Autodesk Fusion 360 part; units mm, degrees
(part 2 of 2)
extrude "Extrude34" add 1 faces at (-31.175, -16.675, -1.0583) along direction (-1, 0, 0) blind 3 separate body on bodies 2 makes body 17
combine "Combine12" operation add target body 2 tool bodies 16 17
combine "Combine13" operation cut target body 2 tool bodies 5 8 4 3 keep tools
sketch "cover" plane through (0, 0, 25) normal (0, 0, 1) x (1, 0, 0)
  line L0 (-31.175, 46.825) -> (-31.175, -48.425)
  line L1 (-31.175, -48.425) -> (-28, -48.425)
  line L2 (-28, -48.425) -> (-28, 46.825)
  line L3 (-28, 46.825) -> (-31.175, 46.825)
  line L4 (-28, 46.825) -> (-28, 40.65)
  line L5 (-28, 40.65) -> (-29.5875, 40.65)
  line L6 (-29.5875, 40.65) -> (27.9875, 40.65)
  line L7 (27.9875, 40.65) -> (27.9875, -45.425)
  line L8 (27.9875, -45.425) -> (-29.5875, -45.425)
  line L9 (-29.5875, -45.425) -> (-29.5875, 40.65)
  dimension "d152" = 6.175
  dimension "d153" = 1.5875
  dimension "d154" = 57.575
  dimension "d155" = 86.075
  constraint coincident L2.end L3.start
  constraint perpendicular L3 L4
  constraint perpendicular L0 L5
  constraint horizontal L6
  constraint vertical L7
  constraint horizontal L8
  constraint vertical L9
  measures "d152" distance of L2.end L4.end
  measures "d153" distance of L4.end L5.end
  measures "d154" distance of L5.end L6.end
  measures "d155" distance of L5.end L8.end
extrude "Extrude35" add sketch "cover" against normal blind 3.175 separate body contours L2 L6 L7 L8 makes body 18
extrude "Extrude36" add 1 faces at (-28, -16.7333, 22.8833) along direction (-1, 0, 0) blind 1.588 separate body on bodies 18 makes body 19
combine "Combine14" operation add target body 18 tool bodies 19
move_body "Move7" bodies 18 to x (1, 0, 0) y (0, 1, 0) z (0, 0, 1) at (0, 0, -3)
extrude "Extrude37" cut 1 faces at (-31.175, 42.7667, 20.7667) along direction (1, 0, 0) blind 3.175 on bodies 8 bodies 8
extrude "Extrude38" cut 1 faces at (29.575, 42.7667, 20.7667) along direction (-1, 0, 0) blind 3.175 on bodies 8 bodies 8
extrude "Extrude39" add 1 faces at (-30.1167, 43.825, 19.5333) along direction (0, -1, 0) blind 3.175 separate body on bodies 5 makes body 20
combine "Combine15" operation add target body 20 tool bodies 5
extrude "Extrude40" add 1 faces at (28.5167, 43.825, 19.5333) along direction (0, -1, 0) blind 3.175 separate body on bodies 4 makes body 21
combine "Combine16" operation add target body 21 tool bodies 4
extrude "Extrude41" add 1 faces at (-30.1167, 42.7667, 6.7) along direction (0, 0, 1) blind 7 on bodies 8 bodies 8
extrude "Extrude42" add 1 faces at (28.5167, 41.7083, 6.7) along direction (0, 0, 1) blind 7 separate body on bodies 8 makes body 22
combine "Combine17" operation add target body 22 tool bodies 8
combine "Combine18" operation cut target body 21 tool bodies 22 keep tools
combine "Combine19" operation cut target body 20 tool bodies 22 keep tools
extrude "Extrude43" add 1 faces at (8.7957, -45.425, 19.8833) along direction (0, -1, 0) blind 3 separate body on bodies 18 makes body 23
combine "Combine20" operation add target body 18 tool bodies 23
combine "Combine21" operation cut target body 20 tool bodies 18 keep tools
combine "Combine22" operation cut target body 21 tool bodies 18 keep tools
sketch "Sketch21" plane through (0, 0, 9.7) normal (0, 0, 1) x (1, 0, 0)
  line L0 (-28, -42.25) -> (-28, -45.425)
  line L1 (-28, -45.425) -> (26.4, -45.425)
  line L2 (26.4, -45.425) -> (26.4, -42.25)
  line L3 (26.4, -42.25) -> (-28, -42.25)
  line L4 (26.4, -45.425) -> (10, -45.425)
  line L5 (10, -45.425) -> (10, -42.25)
  line L6 (10, -42.25) -> (26.4, -42.25)
  line L7 (26.4, -42.25) -> (26.4, -45.425)
  line L8 (-28, -45.425) -> (-10, -45.425)
  line L9 (-10, -45.425) -> (-10, -42.25)
  line L10 (-10, -42.25) -> (-28, -42.25)
  line L11 (-28, -42.25) -> (-28, -45.425)
  dimension "d174" = 16.4
  dimension "d175" = 3.175
  dimension "d176" = 18
  dimension "d177" = 3.175
  constraint horizontal L4
  constraint vertical L5
  constraint horizontal L6
  constraint vertical L7
  constraint coincident L1.end L2.start
  constraint horizontal L8
  constraint vertical L9
  constraint horizontal L10
  constraint vertical L11
  constraint coincident L0.end L1.start
  measures "d174" distance of L1.end L4.end
  measures "d175" distance of L1.end L2.end
  measures "d176" distance of L0.end L8.end
  measures "d177" distance of L0.end L0.start
extrude "Extrude44" add sketch "Sketch21" along normal blind 9.125 separate body contours L0 L1 L3 L8 L9 L10 L11 makes body 24
extrude "Extrude45" add sketch "Sketch21" along normal blind 9.125 separate body contours L1 L2 L3 L4 L5 L6 L7 makes body 25
combine "Combine23" operation add target body 24 tool bodies 3 25
extrude "Extrude46" add 1 faces at (-30.1167, -43.3083, 6.7) along direction (0, 0, 1) blind 5 on bodies 24 bodies 24
extrude "Extrude47" add 1 faces at (28.5167, -44.3667, 6.7) along direction (0, 0, 1) blind 5 on bodies 24 bodies 24
combine "Combine24" operation cut target body 20 tool bodies 24 keep tools
combine "Combine25" operation cut target body 21 tool bodies 24 keep tools
extrude "Extrude48" cut 1 faces at (8.7957, -48.425, 19.8833) along direction (0, 1, 0) blind 3 on bodies 18 bodies 18
sketch "Sketch22" plane through (0, -45.425, 0) normal (0, -1, 0) x (1, 0, 0)
  line L0 (27.9875, 22) -> (-29.588, 22)
  line L1 (-29.588, 22) -> (-29.588, 18.825)
  line L2 (-29.588, 18.825) -> (27.9875, 18.825)
  line L3 (27.9875, 18.825) -> (27.9875, 22)
  line L4 (27.9875, 18.825) -> (9.9995, 18.825)
  line L5 (9.9995, 18.825) -> (-10.0005, 18.825)
  line L6 (-10.0005, 18.825) -> (-10.0005, 22)
  line L7 (-10.0005, 22) -> (9.9995, 22)
  line L8 (9.9995, 22) -> (9.9995, 18.825)
  dimension "d188" = 17.988
  dimension "d189" = 20
  dimension "d190" = 3.175
  constraint coincident L2.end L3.start
  constraint perpendicular L3 L4
  constraint horizontal L5
  constraint vertical L6
  constraint horizontal L7
  constraint vertical L8
  measures "d188" distance of L2.end L4.end
  measures "d189" distance of L4.end L5.end
  measures "d190" distance of L4.end L7.end
extrude "Extrude49" cut sketch "Sketch22" against normal blind 21.6 contours L0 L2 L5 L6 L7 L8 bodies 18
extrude "Extrude50" cut 1 faces at (-3.3338, -23.825, 20.9417) along direction (0, 1, 0) blind 3.175 on bodies 18 bodies 18
extrude "Extrude51" cut 1 faces at (27.4583, 15.075, 25) along direction (0, 0, -1) blind 6.175 on bodies 21 bodies 21
extrude "Extrude52" add 1 faces at (28.5167, 15.075, 18.825) along direction (0, 0, 1) blind 6.175 separate body on bodies 21 makes body 26
combine "Combine26" operation add target body 21 tool bodies 26
extrude "Extrude53" cut 1 faces at (-30.1167, 15.075, 25) along direction (0, 0, -1) blind 6.175 on bodies 20 bodies 20
extrude "Extrude54" add 1 faces at (-30.1167, 15.075, 18.825) along direction (0, 0, 1) blind 6.175 separate body on bodies 20 makes body 27
combine "Combine27" operation add target body 27 tool bodies 20
sketch "lockers" plane through (-31.175, 0, 0) normal (-1, 0, 0) x (0, 0, 1)
  line L0 (11.7, -45.425) -> (3, -45.425)
  line L1 (3, -45.425) -> (3, -42.25)
  line L2 (3, -42.25) -> (11.7, -42.25)
  line L3 (11.7, -42.25) -> (11.7, -45.425)
  line L4 (13.7, 40.65) -> (3, 40.65)
  line L5 (3, 40.65) -> (3, 43.825)
  line L6 (3, 43.825) -> (13.7, 43.825)
  line L7 (13.7, 43.825) -> (13.7, 40.65)
  line L8 (0, -48.425) -> (25, -48.425)
  line L9 (25, -48.425) -> (25, 46.825)
  line L10 (25, 46.825) -> (0, 46.825)
  line L11 (0, 46.825) -> (0, 15)
  line L12 (0, 15) -> (-3.175, 15)
  line L13 (-3.175, 15) -> (-3.175, -15)
  line L14 (-3.175, -15) -> (0, -15)
  line L15 (0, -15) -> (0, -48.425)
  line L16 (0, 0) -> (10, 0)
  line L17 (10, 0) -> (13.175, 0)
  line L18 (13.175, 0) -> (13.175, 5)
  line L19 (13.175, 5) -> (10, 5)
  line L20 (10, 5) -> (10, 0)
  dimension "d203" = 10
  dimension "d204" = 3.175
  dimension "d205" = 5
  constraint coincident L16.start origin
  constraint horizontal L16
  constraint horizontal L17
  constraint vertical L18
  constraint horizontal L19
  constraint vertical L20
  measures "d203" distance of L16.start L16.end
  measures "d204" distance of L16.end L17.end
  measures "d205" distance of L16.end L19.end
extrude "Extrude55" add sketch "lockers" against normal blind 8.175 separate body contours L17 L18 L19 L20 makes body 28
extrude "Extrude56" add 1 faces at (-23, 3.3333, 11.0583) along direction (1, 0, 0) blind 1.6 separate body on bodies 28 makes body 29
combine "Combine28" operation add target body 28 tool bodies 29
combine "Combine29" operation cut target body 27 tool bodies 28 keep tools
copy_body "CopyPasteBodies8" bodies 28 makes body 30
move_body "Move9" bodies 30 to x (1, 0, 0) y (0, 1, 0) z (0, 0, 1) at (50.975, 0, 0)
extrude "Extrude57" cut 1 faces at (19.8, 3.3333, 11.0583) along direction (1, 0, 0) blind 1.6 on bodies 30 bodies 30
combine "Combine30" operation cut target body 21 tool bodies 30 keep tools
extrude "Extrude58" cut 1 faces at (-29.588, -16.7333, 20.9417) along direction (1, 0, 0) blind 1.588 on bodies 18 bodies 18
extrude "Extrude59" cut 1 faces at (27.9875, -16.7333, 20.9417) along direction (-1, 0, 0) blind 1.588 on bodies 18 bodies 18
sketch "Sketch28" plane through (0, 40.65, 0) normal (0, 1, 0) x (-1, 0, 0)
  line L0 (-26.3995, 22) -> (-26.3995, 18.825)
  line L1 (-26.3995, 18.825) -> (28, 18.825)
  line L2 (28, 18.825) -> (28, 22)
  line L3 (28, 22) -> (-26.3995, 22)
  line L4 (-26.3995, 18.825) -> (-21.6995, 18.825)
  line L5 (-21.6995, 18.825) -> (-14.6995, 18.825)
  line L6 (-14.6995, 18.825) -> (-14.6995, 22)
  line L7 (-14.6995, 22) -> (-21.6995, 22)
  line L8 (-21.6995, 22) -> (-21.6995, 18.825)
  line L9 (28, 18.825) -> (21.7, 18.825)
  line L10 (21.7, 18.825) -> (14.7, 18.825)
  line L11 (14.7, 18.825) -> (14.7, 22)
  line L12 (14.7, 22) -> (21.7, 22)
  line L13 (21.7, 22) -> (21.7, 18.825)
  dimension "d216" = 4.7
  dimension "d217" = 7
  dimension "d218" = 3.175
  dimension "d219" = 6.3
  dimension "d220" = 7
  dimension "d221" = 3.175
  constraint coincident L0.end L1.start
  constraint perpendicular L0 L4
  constraint horizontal L5
  constraint vertical L6
  constraint horizontal L7
  constraint vertical L8
  constraint coincident L1.end L2.start
  constraint perpendicular L2 L9
  constraint horizontal L10
  constraint vertical L11
  constraint horizontal L12
  constraint vertical L13
  measures "d216" distance of L0.end L4.end
  measures "d217" distance of L4.end L5.end
  measures "d218" distance of L4.end L7.end
  measures "d219" distance of L1.end L9.end
  measures "d220" distance of L9.end L10.end
  measures "d221" distance of L9.end L12.end
extrude "Extrude60" add sketch "Sketch28" along normal blind 3.175 contours L1 L3 L5 L6 L7 L8 bodies 18
extrude "Extrude61" add sketch "Sketch28" along normal blind 3.175 contours L1 L3 L10 L11 L12 L13 bodies 18
combine "Combine31" operation cut target body 22 tool bodies 18 keep tools
copy_body "CopyPasteBodies9" bodies 2 makes body 31
move_body "Move10" bodies 31 to x (1, 0, 0) y (0, 1, 0) z (0, 0, 1) at (216.211, -13.3874, 0)
sketch "BASE" plane through (0, 0, 0) normal (0, 0, 1) x (1, 0, 0)
  line L0 (206.211, -58.8124) -> (206.211, -55.6374)
  line L1 (206.211, -55.6374) -> (226.211, -55.6374)
  line L2 (226.211, -55.6374) -> (226.211, -58.8124)
  line L3 (226.211, -58.8124) -> (206.211, -58.8124)
  line L4 (245.786, 1.6126) -> (245.786, -28.3874)
  line L5 (245.786, -28.3874) -> (242.611, -28.3874)
  line L6 (242.611, -28.3874) -> (242.611, 1.6126)
  line L7 (242.611, 1.6126) -> (245.786, 1.6126)
  line L8 (206.211, 27.2626) -> (206.211, 30.4376)
  line L9 (206.211, 30.4376) -> (226.211, 30.4376)
  line L10 (226.211, 30.4376) -> (226.211, 27.2626)
  line L11 (226.211, 27.2626) -> (206.211, 27.2626)
  line L12 (188.211, 1.6126) -> (188.211, -28.3874)
  line L13 (188.211, -28.3874) -> (185.036, -28.3874)
  line L14 (185.036, -28.3874) -> (185.036, 1.6126)
  line L15 (185.036, 1.6126) -> (188.211, 1.6126)
  line L16 (248.786, 33.4376) -> (182.036, 33.4376)
  line L17 (182.036, 33.4376) -> (182.036, -61.8124)
  line L18 (182.036, -61.8124) -> (248.786, -61.8124)
  line L19 (248.786, -61.8124) -> (248.786, 33.4376)
copy_body "CopyPasteBodies10" bodies 22 makes body 32
move_body "Move11" bodies 32 to x (1, 0, 0) y (0, 1, 0) z (0, 0, 1) at (124.3455, 0, 4.4249)
sketch "TOP WALL" plane through (0, 40.65, 0) normal (0, -1, 0) x (1, 0, 0)
  line L0 (96.3455, 29.4249) -> (96.3455, 18.1249)
  line L1 (96.3455, 18.1249) -> (93.1705, 18.1249)
  line L2 (93.1705, 18.1249) -> (93.1705, 7.4249)
  line L3 (93.1705, 7.4249) -> (96.3455, 7.4249)
  line L4 (96.3455, 7.4249) -> (96.3455, 4.4249)
  line L5 (96.3455, 4.4249) -> (114.3455, 4.4249)
  line L6 (114.3455, 4.4249) -> (114.3455, 1.2499)
  line L7 (114.3455, 1.2499) -> (134.3455, 1.2499)
  line L8 (134.3455, 1.2499) -> (134.3455, 4.4249)
  line L9 (134.3455, 4.4249) -> (150.7455, 4.4249)
  line L10 (150.7455, 4.4249) -> (150.7455, 7.4249)
  line L11 (150.7455, 7.4249) -> (153.9205, 7.4249)
  line L12 (153.9205, 7.4249) -> (153.9205, 18.1249)
  line L13 (153.9205, 18.1249) -> (150.7455, 18.1249)
  line L14 (150.7455, 18.1249) -> (150.7455, 29.4249)
  line L15 (150.7455, 29.4249) -> (134.3455, 29.4249)
  line L16 (134.3455, 29.4249) -> (134.3455, 14.1249)
  line L17 (134.3455, 14.1249) -> (114.3455, 14.1249)
  line L18 (114.3455, 14.1249) -> (114.3455, 29.4249)
  line L19 (114.3455, 29.4249) -> (96.3455, 29.4249)
  line L20 (102.6455, 23.2499) -> (102.6455, 26.4249)
  line L21 (102.6455, 26.4249) -> (109.6455, 26.4249)
  line L22 (109.6455, 26.4249) -> (109.6455, 23.2499)
  line L23 (109.6455, 23.2499) -> (102.6455, 23.2499)
  line L24 (139.045, 23.2499) -> (139.045, 26.4249)
  line L25 (139.045, 26.4249) -> (146.045, 26.4249)
  line L26 (146.045, 26.4249) -> (146.045, 23.2499)
  line L27 (146.045, 23.2499) -> (139.045, 23.2499)
copy_body "CopyPasteBodies11" bodies 24 makes body 33
move_body "Move12" bodies 33 to x (1, 0, 0) y (0, 1, 0) z (0, 0, 1) at (303.4779, 0, 8.7043)
sketch "BOT WALL" plane through (0, -45.425, 0) normal (0, -1, 0) x (1, 0, 0)
  line L0 (293.4779, 18.4043) -> (293.4779, 27.5293)
  line L1 (293.4779, 27.5293) -> (275.4779, 27.5293)
  line L2 (275.4779, 27.5293) -> (275.4779, 20.4043)
  line L3 (275.4779, 20.4043) -> (272.3029, 20.4043)
  line L4 (272.3029, 20.4043) -> (272.3029, 11.7043)
  line L5 (272.3029, 11.7043) -> (275.4779, 11.7043)
  line L6 (275.4779, 11.7043) -> (275.4779, 8.7043)
  line L7 (275.4779, 8.7043) -> (293.4779, 8.7043)
  line L8 (293.4779, 8.7043) -> (293.4779, 5.5293)
  line L9 (293.4779, 5.5293) -> (313.4779, 5.5293)
  line L10 (313.4779, 5.5293) -> (313.4779, 8.7043)
  line L11 (313.4779, 8.7043) -> (329.8779, 8.7043)
  line L12 (329.8779, 8.7043) -> (329.8779, 11.7043)
  line L13 (329.8779, 11.7043) -> (333.0529, 11.7043)
  line L14 (333.0529, 11.7043) -> (333.0529, 20.4043)
  line L15 (333.0529, 20.4043) -> (329.8779, 20.4043)
  line L16 (329.8779, 20.4043) -> (329.8779, 27.5293)
  line L17 (329.8779, 27.5293) -> (313.4779, 27.5293)
  line L18 (313.4779, 27.5293) -> (313.4779, 18.4043)
  line L19 (313.4779, 18.4043) -> (293.4779, 18.4043)
copy_body "CopyPasteBodies12" bodies 21 makes body 34
move_body "Move13" bodies 34 to x (1, 0, 0) y (0, 1, 0) z (0, 0, 1) at (97.6196, -165.1977, -13.1473)
sketch "RIGHT WALL" plane through (124.0196, 0, 0) normal (-1, 0, 0) x (0, 0, 1)
  line L0 (0.0277, -165.1977) -> (-3.1473, -165.1977)
  line L1 (-3.1473, -165.1977) -> (-3.1473, -160.1977)
  line L2 (-3.1473, -160.1977) -> (0.0277, -160.1977)
  line L3 (0.0277, -160.1977) -> (0.0277, -165.1977)
  line L4 (11.8527, -118.3727) -> (-13.1473, -118.3727)
  line L5 (-13.1473, -118.3727) -> (-13.1473, -150.1977)
  line L6 (-13.1473, -150.1977) -> (-16.3223, -150.1977)
  line L7 (-16.3223, -150.1977) -> (-16.3223, -180.1977)
  line L8 (-16.3223, -180.1977) -> (-13.1473, -180.1977)
  line L9 (-13.1473, -180.1977) -> (-13.1473, -213.6227)
  line L10 (-13.1473, -213.6227) -> (11.8527, -213.6227)
  line L11 (11.8527, -213.6227) -> (11.8527, -118.3727)
  line L12 (-10.1473, -124.5477) -> (-10.1473, -121.3727)
  line L13 (-10.1473, -121.3727) -> (0.5527, -121.3727)
  line L14 (0.5527, -121.3727) -> (0.5527, -124.5477)
  line L15 (0.5527, -124.5477) -> (-10.1473, -124.5477)
  line L16 (-1.4473, -207.4477) -> (-1.4473, -210.6227)
  line L17 (-1.4473, -210.6227) -> (-10.1473, -210.6227)
  line L18 (-10.1473, -210.6227) -> (-10.1473, -207.4477)
  line L19 (-10.1473, -207.4477) -> (-1.4473, -207.4477)
copy_body "CopyPasteBodies13" bodies 27 makes body 35
move_body "Move14" bodies 35 to x (1, 0, 0) y (0, 1, 0) z (0, 0, 1) at (0, 159.0386, 7.9675)
sketch "LEFT WALL" plane through (-31.175, 0, 0) normal (-1, 0, 0) x (0, 0, 1)
  line L0 (21.1425, 159.0386) -> (17.9675, 159.0386)
  line L1 (17.9675, 159.0386) -> (17.9675, 164.0386)
  line L2 (17.9675, 164.0386) -> (21.1425, 164.0386)
  line L3 (21.1425, 164.0386) -> (21.1425, 159.0386)
  line L4 (19.6675, 113.6136) -> (10.9675, 113.6136)
  line L5 (10.9675, 113.6136) -> (10.9675, 116.7886)
  line L6 (10.9675, 116.7886) -> (19.6675, 116.7886)
  line L7 (19.6675, 116.7886) -> (19.6675, 113.6136)
  line L8 (21.6675, 199.6886) -> (10.9675, 199.6886)
  line L9 (10.9675, 199.6886) -> (10.9675, 202.8636)
  line L10 (10.9675, 202.8636) -> (21.6675, 202.8636)
  line L11 (21.6675, 202.8636) -> (21.6675, 199.6886)
  line L12 (7.9675, 110.6136) -> (32.9675, 110.6136)
  line L13 (32.9675, 110.6136) -> (32.9675, 205.8636)
  line L14 (32.9675, 205.8636) -> (7.9675, 205.8636)
  line L15 (7.9675, 205.8636) -> (7.9675, 174.0386)
  line L16 (7.9675, 174.0386) -> (4.7925, 174.0386)
  line L17 (4.7925, 174.0386) -> (4.7925, 144.0386)
  line L18 (4.7925, 144.0386) -> (7.9675, 144.0386)
  line L19 (7.9675, 144.0386) -> (7.9675, 110.6136)
copy_body "CopyPasteBodies14" bodies 18 makes body 36
move_body "Move15" bodies 36 to x (1, 0, 0) y (0, 1, 0) z (0, 0, 1) at (-156.7404, 0, -13.2817)
sketch "COVER" plane through (0, 0, 8.7183) normal (0, 0, 1) x (1, 0, 0)
  line L0 (-130.3409, -45.425) -> (-130.3409, 40.65)
  line L1 (-130.3409, 40.65) -> (-135.0409, 40.65)
  line L2 (-135.0409, 40.65) -> (-135.0409, 43.825)
  line L3 (-135.0409, 43.825) -> (-142.0409, 43.825)
  line L4 (-142.0409, 43.825) -> (-142.0409, 40.65)
  line L5 (-142.0409, 40.65) -> (-171.4404, 40.65)
  line L6 (-171.4404, 40.65) -> (-171.4404, 43.825)
  line L7 (-171.4404, 43.825) -> (-178.4404, 43.825)
  line L8 (-178.4404, 43.825) -> (-178.4404, 40.65)
  line L9 (-178.4404, 40.65) -> (-184.7404, 40.65)
  line L10 (-184.7404, 40.65) -> (-184.7404, -45.425)
  line L11 (-184.7404, -45.425) -> (-166.7409, -45.425)
  line L12 (-166.7409, -45.425) -> (-166.7409, -20.65)
  line L13 (-166.7409, -20.65) -> (-146.7409, -20.65)
  line L14 (-146.7409, -20.65) -> (-146.7409, -45.425)
  line L15 (-146.7409, -45.425) -> (-130.3409, -45.425)
copy_body "CopyPasteBodies15" bodies 28 makes body 37
move_body "Move16" bodies 37 to x (1, 0, 0) y (0, 1, 0) z (0, 0, 1) at (0, -118.2751, -5.7778)
sketch "LOCKER1" plane through (0, 0, 7.3972) normal (0, 0, 1) x (1, 0, 0)
  line L0 (-31.175, -113.2751) -> (-31.175, -118.2751)
  line L1 (-31.175, -118.2751) -> (-21.4, -118.2751)
  line L2 (-21.4, -118.2751) -> (-21.4, -113.2751)
  line L3 (-21.4, -113.2751) -> (-31.175, -113.2751)
copy_body "CopyPasteBodies16" bodies 30 makes body 38
move_body "Move17" bodies 38 to x (1, 0, 0) y (0, 1, 0) z (0, 0, 1) at (8.0146, -133.5287, 0)
sketch "LOCKER2" plane through (0, 0, 13.175) normal (0, 0, 1) x (1, 0, 0)
  line L0 (29.4146, -128.5287) -> (29.4146, -133.5287)
  line L1 (29.4146, -133.5287) -> (37.5896, -133.5287)
  line L2 (37.5896, -133.5287) -> (37.5896, -128.5287)
  line L3 (37.5896, -128.5287) -> (29.4146, -128.5287)
hidden bodies 31 32 33 34 35 36 37 38
equation "d36 = ( -2.54 * 4 ) * 1 mm"
equation "d37 = ( 2.54 * 14 ) * 1 mm"
equation "d43 = ( 2.54 * 2 ) * 1 mm"
equation "d47 = ( 12 * 2.54 ) * 1 mm"
equation "d52 = ( 2.54 * 3 / 5 ) * 1 mm"
equation "d55 = ( 2.54 * 3 / 5 ) * 1 mm"
named bodies: "bb", "base", "bot wall", "right wall", "left wall", "top wall", "cover", "locker1", "locker2", "base (1)", "top wall (1)", "bot wall (1)", "right wall (1)", "left wall (1)", "cover (1)", "locker1 (1)", "locker2 (1)"
